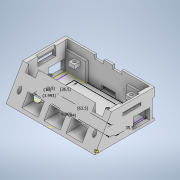
# Autodesk Inventor part: Base Onixium
Saved by Autodesk Inventor 2021 (Build 250183000, 183)
## iProperties
Created: 2021-10-26
Part Number: Base Onixium
Material: Genérico
Document SubType Name: Chapa
Designer: Juan Camilo
Density: 1 g/cm^3
Sheet Metal Rule: Por defecto_mm
Appearance: Valor por defecto
Author: Juan Camilo
Autodesk Inventor part; units mm, degrees
ref_plane "YZ Plane" through (0, 0, 0) normal (1, 0, 0) x (0, 1, 0)
ref_plane "XZ Plane" through (0, 0, 0) normal (0, 1, 0) x (-1, 0, 0)
ref_plane "XY Plane" through (0, 0, 0) normal (0, 0, 1) x (1, 0, 0)
sketch "Boceto2" plane through (0, 0, 0) normal (0, 1, 0) x (-1, 0, 0)
  line L0 (-49, 0) -> (49, 0)
  line L1 (49, 0) -> (49, -87)
  line L2 (49, -87) -> (-49, -87)
  line L3 (-49, -87) -> (-49, 0)
  line L4 (0, -87) -> (0, 0) construction
  circle A0 centre (-41.5, -7.5) radius 1.75
  circle A1 centre (41.5, -7.5) radius 1.75
  line L5 (-26, -87) -> (-26, -66)
  line L6 (-26, -66) -> (-49, -66)
  line L7 (26, -87) -> (26, -66)
  line L8 (26, -66) -> (49, -66)
  line L9 (49, -12) -> (-49, -12) construction
  line L10 (44.5, -24.05) -> (28.5, -24.05)
  line L11 (28.5, -24.05) -> (28.5, -13.05)
  line L12 (28.5, -13.05) -> (44.5, -13.05)
  line L13 (44.5, -13.05) -> (44.5, -24.05)
  line L14 (42.5, -23.55) -> (31.5, -23.55)
  line L15 (31.5, -14.85) -> (42.5, -14.85)
  line L16 (42.5, -14.85) -> (42.5, -23.55)
  circle A2 centre (30.2, -19.25) radius 1.05
  line L17 (31.5, -14.85) -> (31.5, -23.55)
  line L18 (-42.5, -23.55) -> (-31.5, -23.55)
  line L19 (-31.5, -14.85) -> (-42.5, -14.85)
  line L20 (-42.5, -14.85) -> (-42.5, -23.55)
  circle A3 centre (-30.2, -19.25) radius 1.05
  line L21 (-31.5, -14.85) -> (-31.5, -23.55)
  circle A4 centre (13, -21.5) radius 2.5
  circle A5 centre (-13, -21.5) radius 2.5
  circle A6 centre (16, -70) radius 2.5
  circle A7 centre (-16, -70) radius 2.5
  point P0 (26, -87)
  dimension "d6" = 3.5
  dimension "d210" = 0
  dimension "d219" = 87
  dimension "d220" = 21
  dimension "d221" = 12
  dimension "d222" = 23
  dimension "d223" = 98
  dimension "d224" = 7.5
  dimension "d225" = 7.5
  dimension "d226" = 79.5
  dimension "d229" = 2.1
  dimension "d230" = 9
  dimension "d231" = 11
  dimension "d232" = 16
  dimension "d235" = 1
  dimension "d236" = 3.6
  dimension "d239" = 2.1
  dimension "d241" = 1.3
  dimension "d242" = 5
  dimension "d243" = 36
  dimension "d244" = 9.5
  dimension "d245" = 5
  dimension "d246" = 17
  dimension "d247" = 10
  dimension "d252" = 8.7
  dimension "d254" = 4.3
  dimension "d255" = 4
  dimension "d256" = 11
  dimension "d257" = 54
  dimension "d258" = 2.85
  constraints: 44 end point, 10 symmetric about line, 8 centre point, 5 parallel, 5 point on line, 4 horizontal, 4 perpendicular, 3 midpoint, 1 equal radius, 1 vertical, 3 other
  measures "d6" diameter of A0
  measures "d210" distance of point (0, 0) L4.end
  measures "d219" distance of L1.start L1.end
  measures "d220" distance of L7.start L8.start
  measures "d221" distance between parallel lines of L0 L9
  measures "d222" distance of L8.start L8.end
  measures "d223" distance of L0.start L1.start
  measures "d224" distance from line of L1 A1.centre
  measures "d225" distance from line of L0 A1.centre
  measures "d229" diameter of L9 L12
  measures "d230" diameter of L1 L13
  measures "d231" distance of L10.end L11.end
  measures "d232" distance of L10.start L10.end
  measures "d235" diameter of L14 L10
  measures "d236" diameter of L15 L12
  measures "d239" diameter of A2
  measures "d241" distance from line of L17 A2.centre
  measures "d242" diameter of A4
  measures "d243" distance from line of L1 A4.centre
  measures "d244" distance from line of L9 A4.centre
  measures "d245" diameter of A6
  measures "d246" distance from line of L2 A6.centre
  measures "d247" distance from line of L7 A6.centre
  measures "d252" distance of L15.start L14.end
  measures "d254" distance from line of L14 A2.centre
  measures "d255" diameter of L16 L13
  measures "d256" distance of L15.start L15.end
  measures "d257" distance between parallel lines of L9 L8
  measures "d258" distance between parallel lines of L9 L15
extrude "Extrusion Base" add sketch "Boceto2" along normal blind 2 contours L0 L1 L8 L7 L2 L5 L6 L3 | L10 L11 L12 L13
sketch "Boceto4" plane through (-49, 0, -66) normal (-1, 0, 0) x (0, 0, 1)
  line L0 (66, 0) -> (0, 0) projected
  line L1 (66, 0) -> (64.8476, 2)
  line L2 (66, 0) -> (68.3082, 0) construction
  line L3 (64.8476, 2) -> (66, 2)
  line L4 (66, 0) -> (66, 2) projected
  line L5 (66, 2) -> (66, 0)
  dimension "d24" = 119.95
  constraints: 8 end point, 2 horizontal, 1 equal length, 1 perpendicular
  measures "d24" angle of L2 L1
extrude "Extrusión Angulo parte de adelante" cut sketch "Boceto4" against normal blind 100
sketch "Boceto5" plane through (0, 2, 0) normal (0, 1, 0) x (1, 0, 0)
  line L0 (49, 66) -> (26, 66) projected
  line L1 (-49, 66) -> (-49, 1.1524) projected
  line L2 (49, 66) -> (-49, 66)
  line L3 (-49, 66) -> (-49, 61.5)
  line L4 (-49, 61.5) -> (49, 61.5)
  line L5 (49, 61.5) -> (49, 66)
  point P0 (0, 0)
  dimension "d27" = 4.5
  constraints: 8 end point, 2 parallel, 1 horizontal, 1 perpendicular, 1 point on line
  measures "d27" distance of L3.end L2.end
extrude "parte trasera diseño" add sketch "Boceto5" along normal blind 30
sketch "Boceto6" plane through (-26, 0, -66) normal (0, 0, -1) x (-1, 0, 0)
  line L0 (23, 0) -> (23, 32) projected
  line L1 (23, 0) -> (23, 3.33)
  line L2 (23, 3.33) -> (0, 3.33)
  line L3 (0, 3.33) -> (0, 22.33)
  line L4 (0, 22.33) -> (23, 22.33)
  line L5 (23, 22.33) -> (23, 3.33)
  line L6 (-26, 0) -> (-26, 32)
  line L7 (-75, 32) -> (23, 32) projected
  line L8 (-52, 3.33) -> (-52, 22.33)
  line L9 (-52, 22.33) -> (-75, 22.33)
  line L10 (-75, 3.33) -> (-52, 3.33)
  line L11 (-75, 0) -> (-75, 32)
  line L12 (-75, 22.33) -> (-75, 3.33)
  dimension "d30" = 3.33
  dimension "d31" = 23
  dimension "d32" = 19
  constraints: 22 end point, 5 symmetric about line, 2 parallel, 2 point on line, 1 horizontal, 1 midpoint, 1 perpendicular
  measures "d30" distance of L0.start L1.end
  measures "d31" distance of L3.end L4.end
  measures "d32" distance of L2.end L3.end
extrude "Extrusión parte trasera diseño con empalmes" cut sketch "Boceto6" against normal blind 2.5
fillet "Empalme parte trasera diseño" radius 2 4 edges at (-37.5, 22.33, -66) (-37.5, 3.33, -66) (37.5, 3.33, -66) (37.5, 22.33, -66)
sketch "Boceto7" plane through (0, 32, 0) normal (0, 1, 0) x (1, 0, 0)
  line L0 (49, 61.5) -> (49, 66) projected
  line L1 (49, 61.5) -> (22.385, 61.5)
  line L2 (22.385, 61.5) -> (22.385, 64)
  line L3 (22.385, 64) -> (49, 64)
  line L4 (49, 64) -> (49, 61.5)
  line L5 (49, 61.5) -> (-49, 61.5) projected
  line L6 (0, 61.5) -> (0, 0)
  line L7 (-49, 61.5) -> (-49, 66)
  line L8 (-49, 61.5) -> (-22.385, 61.5)
  line L9 (-22.385, 61.5) -> (-22.385, 64)
  line L10 (-22.385, 64) -> (-49, 64)
  line L11 (-22.385, 61.5) -> (22.385, 61.5)
  line L12 (22.385, 61.5) -> (22.385, 64)
  line L13 (22.385, 64) -> (-22.385, 64)
  line L14 (-22.385, 64) -> (-22.385, 61.5)
  dimension "d36" = 26.615
  dimension "d37" = 2.5
  constraints: 26 end point, 4 parallel, 4 symmetric about line, 2 horizontal, 2 perpendicular, 1 midpoint, 1 vertical
  measures "d36" distance of L2.end L3.end
  measures "d37" distance of L1.end L2.end
extrude "Parte delantera de la parte trasera diseño" cut sketch "Boceto7" against normal blind 30 contours L5 L9 L13 L2
sketch "Boceto8" plane through (22.385, 32, -64) normal (-1, 0, 0) x (0, 0, 1)
  line L0 (2.5, 0) -> (2.5, -30) projected
  line L1 (2.5, -30) -> (0, -30)
  line L2 (0, -30) -> (0, -9)
  line L3 (0, -9) -> (2.5, -9)
  line L4 (2.5, -9) -> (2.5, -30)
  line L5 (0, 0) -> (2.5, 0) projected
  line L6 (2.5, -9) -> (0, -9)
  line L7 (0, -9) -> (0, 0)
  line L8 (0, 0) -> (2.5, 0)
  line L9 (2.5, 0) -> (2.5, -9)
  point P0 (64, -32)
  point P1 (0, -9)
  point P2 (2.5, -9)
  dimension "d40" = 2.5
  dimension "d41" = 21
  constraints: 16 end point, 4 parallel, 2 horizontal, 2 perpendicular
  measures "d40" distance of L2.end L3.end
  measures "d41" distance of L1.end L2.end
extrude "Extrusión Parte delantera de la parte trasera del diseño" cut sketch "Boceto8" along normal blind 67.77 and the other way blind 23.15 contours L0 L3 L7 L5
sketch "Boceto9" plane through (0, 32, 0) normal (0, 1, 0) x (1, 0, 0)
  line L0 (49, 0) -> (49, 66) projected
  line L1 (49, 66) -> (15, 66)
  line L2 (49, 66) -> (-49, 66) projected
  line L3 (15, 66) -> (5, 66)
  line L4 (5, 66) -> (5, 64)
  line L5 (5, 64) -> (15, 64)
  line L6 (15, 64) -> (15, 66)
  line L7 (0, 66) -> (0, 64)
  line L8 (-45.385, 64) -> (45.535, 64) projected
  line L9 (-49, 66) -> (49, 66)
  line L10 (-15, 66) -> (-5, 66)
  line L11 (-5, 66) -> (-5, 64)
  line L12 (-5, 64) -> (-15, 64)
  line L13 (-15, 64) -> (-15, 66)
  point P0 (0, 0)
  point P1 (-15, 64)
  point P2 (-5, 64)
  dimension "d46" = 34
  dimension "d47" = 10
  dimension "d48" = 2
  dimension "d49" = 2
  constraints: 22 end point, 6 symmetric about line, 3 point on line, 2 parallel, 1 horizontal, 1 midpoint, 1 perpendicular
  measures "d46" distance of L0.end L1.end
  measures "d47" distance of L5.end L4.end
  measures "d48" distance of L4.end L3.end
  measures "d49" distance of L7.start L7.end
extrude "Extrusión Parte Trasera De la Parte trasera diseño" cut sketch "Boceto9" against normal blind 4 contours L6 L5 L4 L2 | L11 L8 L13 L2
sketch "Boceto10" plane through (49, 0, 0) normal (1, 0, 0) x (0, 0, -1)
  line L0 (0, 0) -> (1.1524, 2) projected
  line L1 (1.1524, 2) -> (0, 2)
  line L2 (61.5, 32) -> (66, 32) projected
  line L3 (0, 2) -> (61.5, 2)
  line L4 (61.5, 2) -> (61.5, 32)
  line L5 (61.5, 32) -> (0, 32)
  line L6 (0, 32) -> (0, 2)
  point P0 (1.1524, 2)
  constraints: 10 end point, 2 horizontal, 2 parallel, 1 perpendicular
extrude "Grado de inclinacion de 60.5 de parte delantera" add sketch "Boceto10" against normal blind 4
sketch "Boceto11" plane through (-49, 0, -66) normal (-1, 0, 0) x (0, 0, 1)
  line L0 (64.8476, 2) -> (4.5, 2) projected
  line L1 (64.8476, 2) -> (66, 2) projected
  line L2 (66, 2) -> (66, 32) projected
  line L3 (66, 32) -> (4.5, 32) projected
  line L4 (4.5, 32) -> (4.5, 23) projected
  line L5 (4.5, 2) -> (4.5, 23) projected
  line L6 (4.5, 2) -> (4.5, 32) projected
  line L7 (66, 2) -> (4.5, 2)
  line L8 (4.5, 2) -> (4.5, 32)
  line L9 (4.5, 32) -> (66, 32)
  line L10 (66, 32) -> (66, 2)
  point P0 (66, 0)
  point P1 (4.5, 2)
  constraints: 8 end point, 2 parallel, 1 horizontal, 1 perpendicular
extrude "Lateral derecha de diseño" add sketch "Boceto11" against normal blind 4
sketch "Boceto12" plane through (0, 32, 0) normal (0, 1, 0) x (1, 0, 0)
  line L0 (45, 0) -> (-45, 0)
  line L1 (-45, 0) -> (-45, 4)
  line L2 (-45, 4) -> (45, 4)
  line L3 (45, 4) -> (45, 0)
  line L4 (0, 4) -> (0, 64)
  line L5 (-5, 64) -> (5, 64) projected
  point P0 (0, 0)
  point P1 (-45, 0)
  point P2 (-49, 0)
  dimension "d56" = 4
  constraints: 10 end point, 2 midpoint, 2 parallel, 1 horizontal, 1 perpendicular
  measures "d56" distance of L0.end L1.end
extrude "Parte delantera diseño" add sketch "Boceto12" against normal blind 30
sketch "Boceto13" plane through (49, 0, 0) normal (1, 0, 0) x (0, 0, -1)
  line L0 (1.1524, 2) -> (0, 0) projected
  line L1 (0, 0) -> (18.438, 32)
  line L2 (0, 32) -> (61.5, 32) projected
  line L3 (0, 0) -> (36.9318, 0) construction
  line L4 (18.438, 32) -> (0, 32)
  line L5 (0, 32) -> (0, 0)
  point P0 (4, 32)
  point P1 (1.1524, 2)
  point P2 (4, 32)
  dimension "d59" = 60.05
  constraints: 8 end point, 1 collinear, 1 equal length, 1 horizontal, 1 perpendicular, 1 point on line
  measures "d59" angle of L3 L1
extrude "Lateral izquierda diseño" cut sketch "Boceto13" against normal blind 103.25
sketch "Boceto14" plane through (26, 0, -66) normal (1, 0, 0) x (0, 0, -1)
  line L0 (21, 2) -> (0, 2) projected
  line L1 (21, 2) -> (19.5, 0)
  line L2 (21, 2) -> (23.5, 2) construction
  line L3 (21, 0) -> (0, 0) projected
  line L4 (19.5, 0) -> (21, 0)
  line L5 (21, 0) -> (21, 2) projected
  line L6 (21, 0) -> (21, 2)
  point P0 (-66, 0)
  point P1 (19.5, 0)
  dimension "d62" = 126.87
  constraints: 8 end point, 1 collinear, 1 equal length, 1 horizontal, 1 perpendicular
  measures "d62" angle of L1 L2
extrude "Extrusion para placa trasera" cut sketch "Boceto14" against normal blind 57.5
sketch "Boceto15" plane through (-45, 0, -66) normal (1, 0, 0) x (0, 0, -1)
  line L0 (-47.562, 32) -> (-66, 0) projected
  line L1 (-66, 0) -> (0, 0) projected
  line L2 (0, 0) -> (0, 1.33) projected
  arc A0 (0, 1.33) -> (-2, 3.33) centre (-2, 1.33) ccw projected
  line L3 (-2, 3.33) -> (-2.5, 3.33) projected
  line L4 (-2.5, 3.33) -> (-2.5, 22.33) projected
  line L5 (-2.5, 22.33) -> (-2, 22.33) projected
  arc A1 (-2, 22.33) -> (0, 24.33) centre (-2, 24.33) ccw projected
  line L6 (0, 24.33) -> (0, 32) projected
  line L7 (0, 32) -> (-47.562, 32) projected
  line L8 (-4.5, 32) -> (-47.562, 32) projected
  line L9 (-47.562, 32) -> (-47.562, 0)
  line L10 (0, 0) -> (-66, 0) projected
  line L11 (-66, 0) -> (-47.562, 32) projected
  line L12 (-66, 0) -> (-47.562, 0)
  line L13 (-66, 0) -> (-47.562, 32)
  constraints: 6 end point, 1 collinear, 1 point on line, 1 vertical
extrude "Extrusion capa parte delantera" add sketch "Boceto15" along normal blind 93 contours L9 L1 L0
sketch "Boceto17" plane through (0, 0, 0) normal (0, -1, 0) x (1, 0, 0)
  line L0 (-49, 0) -> (49, 0) projected
  line L1 (49, 0) -> (41.5, 0)
  line L2 (41.5, 0) -> (41.5, -7.5)
  line L3 (41.5, -7.5) -> (49, -7.5)
  line L4 (49, -7.5) -> (49, 0)
  circle A0 centre (41.5, -7.5) radius 1.75
  line L5 (0, 0) -> (0, -85.5)
  line L6 (-26, -85.5) -> (26, -85.5) projected
  circle A1 centre (-41.5, -7.5) radius 1.75
  dimension "d67" = 7.5
  dimension "d68" = 7.5
  dimension "d69" = 3.5
  constraints: 10 end point, 2 centre point, 2 parallel, 1 coincident, 1 horizontal, 1 midpoint, 1 perpendicular, 1 symmetric about line, 1 other
  measures "d67" distance of L3.end L2.end
  measures "d68" distance of L2.end L1.end
  measures "d69" diameter of A0
extrude "Extrusión huecos tornillos parte delantera" cut sketch "Boceto17" against normal blind 90.25 contours A0 L3 L2 | L2 L3 A0 | A1
sketch "Boceto24" plane through (0, 2, 0) normal (0, 1, 0) x (1, 0, 0)
  line L0 (45.535, 61.5) -> (45, 61.5) projected
  line L1 (45, 61.5) -> (32, 61.5)
  line L2 (32, 61.5) -> (32, 31.5)
  line L3 (32, 31.5) -> (45, 31.5)
  line L4 (45, 31.5) -> (45, 61.5)
  circle A0 centre (32, 31.5) radius 1.75
  circle A1 centre (32, 31.5) radius 2.25
  line L5 (-5, 64) -> (5, 64) projected
  line L6 (0, 64) -> (0, 39.9317)
  circle A2 centre (-32, 31.5) radius 1.75
  circle A3 centre (-32, 31.5) radius 2.25
  point P0 (0, 0)
  dimension "d120" = 13
  dimension "d121" = 30
  dimension "d122" = 3.5
  dimension "d123" = 4.5
  dimension "d143" = 59.5
  constraints: 10 end point, 4 centre point, 3 coincident, 2 parallel, 2 symmetric about line, 1 horizontal, 1 midpoint, 1 perpendicular, 1 vertical, 2 other
  measures "d120" distance of L3.end L2.end
  measures "d121" distance of L2.end L1.end
  measures "d122" diameter of A0
  measures "d123" diameter of A1
extrude "Tornillos Placa" add sketch "Boceto24" along normal blind 18 contours A1 L3 A0 L2 | L2 A0 L3 A1 | A3
thread "Rosca1" size "M3.5x0.6" class "6H" standard "ANSI Metric M Profile" full length
thread "Rosca2" size "M3.5x0.6" class "6H" standard "ANSI Metric M Profile" full length
sketch "Boceto25" plane through (-49, 0, -66) normal (-1, 0, 0) x (0, 0, 1)
  line L0 (5.5, 15) -> (23.5, 15)
  line L1 (23.5, 15) -> (23.5, 3)
  line L2 (23.5, 3) -> (5.5, 3)
  line L3 (5.5, 3) -> (5.5, 15)
  line L4 (2.5, 22.33) -> (2.5, 3.33) projected
  line L5 (0, 0) -> (66, 0) projected
  dimension "d130" = 3
  dimension "d131" = 3
  dimension "d132" = 18
  dimension "d133" = 12
  constraints: 8 end point, 2 parallel, 1 horizontal, 1 perpendicular
  measures "d130" distance between parallel lines of L4 L3
  measures "d131" distance between parallel lines of L5 L2
  measures "d132" distance of L0.start L0.end
  measures "d133" distance of L0.end L1.end
extrude "Extrusión sensores laterales" cut sketch "Boceto25" against normal blind 98.25
sketch "Boceto26" plane through (26, 2, -66) normal (0, 0, -1) x (-1, 0, 0)
  line L0 (18.5, 5) -> (33.5, 5)
  line L1 (33.5, 5) -> (33.5, 0)
  line L2 (33.5, 0) -> (18.5, 0)
  line L3 (18.5, 0) -> (18.5, 5)
  line L4 (52, 0) -> (0, 0) projected
  line L5 (52, 0) -> (52, 22.33) projected
  line L6 (0, 0) -> (0, 22.33) projected
  point P0 (26, -2)
  dimension "d136" = 15
  dimension "d137" = 5
  dimension "d138" = 0
  dimension "d139" = 18.5
  dimension "d140" = 18.5
  constraints: 8 end point, 2 parallel, 1 horizontal, 1 perpendicular
  measures "d136" distance of L0.start L0.end
  measures "d137" distance of L2.end L0.start
  measures "d138" distance between parallel lines of L4 L2
  measures "d139" distance between parallel lines of L5 L1
  measures "d140" distance between parallel lines of L6 L3
extrude "Extrusión agujero cables inferiores" cut sketch "Boceto26" against normal blind 3
sketch "Boceto27" plane through (-45, 2, -18.438) normal (0, 0, -1) x (-1, 0, 0)
  line L0 (-78.5, 13) -> (-60.5, 13)
  line L1 (-60.5, 13) -> (-60.5, 1)
  line L2 (-60.5, 1) -> (-78.5, 1)
  line L3 (-78.5, 1) -> (-78.5, 13)
  line L4 (0, 0) -> (-90, 0) projected
  line L5 (-90, 0) -> (-90, 30) projected
  line L6 (-54.1, 13) -> (-36.1, 13)
  line L7 (-36.1, 13) -> (-36.1, 1)
  line L8 (-36.1, 1) -> (-54.1, 1)
  line L9 (-54.1, 1) -> (-54.1, 13)
  line L10 (-29.7, 13) -> (-11.7, 13)
  line L11 (-11.7, 13) -> (-11.7, 1)
  line L12 (-11.7, 1) -> (-29.7, 1)
  line L13 (-29.7, 1) -> (-29.7, 13)
  point P0 (-45, -2)
  point P1 (-13.5, 0)
  point P2 (-76.5, 0)
  dimension "d144" = 18
  dimension "d145" = 12
  dimension "d146" = 1
  dimension "d147" = 11.5
  dimension "d148" = 1
  dimension "d149" = 12
  dimension "d150" = 18
  dimension "d151" = 6.4
  dimension "d152" = 6.4
  dimension "d153" = 1
  dimension "d154" = 18
  dimension "d155" = 12
  constraints: 24 end point, 6 parallel, 3 horizontal, 3 perpendicular
  measures "d144" distance of L0.start L0.end
  measures "d145" distance of L0.end L1.end
  measures "d146" distance between parallel lines of L4 L2
  measures "d147" distance between parallel lines of L5 L3
  measures "d148" distance between parallel lines of L4 L8
  measures "d149" distance of L8.end L6.start
  measures "d150" distance of L6.start L6.end
  measures "d151" distance between parallel lines of L9 L1
  measures "d152" distance between parallel lines of L7 L13
  measures "d153" distance between parallel lines of L4 L12
  measures "d154" distance of L10.start L10.end
  measures "d155" distance of L10.end L11.end
extrude "Extrusión sensores delanteros" cut sketch "Boceto27" against normal blind 19.25
sketch "Boceto28" plane through (-22.385, 2, -61.5) normal (0, 0, 1) x (1, 0, 0)
  line L0 (-12.615, 14) -> (-5.615, 14)
  line L1 (-5.615, 14) -> (-5.615, 18)
  line L2 (-5.615, 18) -> (-12.615, 18)
  line L3 (-12.615, 18) -> (-12.615, 14)
  line L4 (0, 0) -> (-22.615, 0) projected
  line L5 (-22.615, 21) -> (-22.615, 0) projected
  line L6 (22.385, -2) -> (22.385, 31.9246)
  line L7 (57.385, 14) -> (50.385, 14)
  line L8 (50.385, 14) -> (50.385, 18)
  line L9 (50.385, 18) -> (57.385, 18)
  line L10 (57.385, 18) -> (57.385, 14)
  dimension "d158" = 18
  dimension "d159" = 4
  dimension "d160" = 7
  dimension "d161" = 10
  constraints: 18 end point, 4 symmetric about line, 2 parallel, 1 horizontal, 1 perpendicular, 1 vertical
  measures "d158" distance between parallel lines of L4 L2
  measures "d159" distance between parallel lines of L0 L2
  measures "d160" distance of L1.end L2.end
  measures "d161" distance between parallel lines of L5 L3
extrude "Extrusión pads tornillos traseros placa" add sketch "Boceto28" along normal blind 7
sketch "Boceto29" plane through (-35, 20, -61.5) normal (0, 1, 0) x (1, 0, 0)
  line L0 (7, -7) -> (0, -7) projected
  line L1 (3.5, -7) -> (3.5, 1.276)
  line L2 (0, 0) -> (0, -7) projected
  line L3 (0, -3.5) -> (7, -3.5)
  line L4 (7, 0) -> (7, -7) projected
  circle A0 centre (3.5, -3.5) radius 1.75
  line L5 (35, 2.507) -> (35, -61.5)
  circle A1 centre (66.5, -3.5) radius 1.75
  dimension "d164" = 3.5
  constraints: 6 end point, 4 midpoint, 2 centre point, 2 vertical, 1 symmetric about line, 1 other
  measures "d164" diameter of A0
extrude "Extrusión tornillos" cut sketch "Boceto29" against normal blind 4.75 contours A0 L3 L1 | L1 L3 A0 | L3 L1 A0 | L3 A0 L1 | A1
sketch "Boceto placa" plane through (0, 2, 0) normal (0, 1, 0) x (1, 0, 0)
  circle A0 centre (-32, 31.5) radius 1.75 projected
  circle A1 centre (31.5, 58) radius 1.75 projected
  line L0 (-32, 31.5) -> (31.5, 31.5)
  line L1 (31.5, 31.5) -> (31.5, 58)
  line L2 (31.5, 58) -> (-32, 58)
  line L3 (-32, 58) -> (-32, 31.5)
  line L4 (-42, 27.507) -> (42, 27.507)
  line L5 (42, 27.507) -> (42, 63.007)
  line L6 (42, 63.007) -> (-42, 63.007)
  line L7 (-42, 63.007) -> (-42, 27.507)
  line L8 (-45, 61.5) -> (-45, 18.438) projected
  line L9 (45, 18.438) -> (45, 61.5) projected
  line L10 (-22.385, 61.5) -> (-45, 61.5) projected
  line L11 (-44, 25.3) -> (-33.55, 25.3) projected
  line L12 (-45, 18.438) -> (45, 18.438) projected
  point P0 (0, 0)
  dimension "d167" = 63.5
  dimension "d168" = 26.5
  dimension "d172" = 84
  dimension "d176" = 10
  dimension "d177" = 3.993
  dimension "d178" = 3.5
  dimension "d179" = 35.5
  dimension "d180" = 9.069
  constraints: 16 end point, 4 parallel, 2 horizontal, 2 perpendicular
  measures "d167" distance of L0.start L0.end
  measures "d168" distance of L2.end L0.start
  measures "d172" distance of L4.start L4.end
  measures "d176" distance from line of L7 L0.start
  measures "d177" distance from line of L4 L0.start
  measures "d178" diameter of A0
  measures "d179" distance between parallel lines of L6 L4
  measures "d180" distance between parallel lines of L12 L4
sketch "Boceto32" plane through (0, 32, 0) normal (0, 1, 0) x (1, 0, 0)
  line L0 (45, 31) -> (47, 31)
  line L1 (47, 31) -> (47, 51)
  line L2 (47, 51) -> (45, 51)
  line L3 (45, 51) -> (45, 31)
  line L4 (49, 66) -> (15, 66) projected
  line L5 (45, 18.438) -> (49, 18.438) projected
  line L6 (49, 66) -> (49, 18.438) projected
  line L7 (0, 0) -> (0, 66)
  line L8 (5, 66) -> (-5, 66) projected
  line L9 (-45, 31) -> (-47, 31)
  line L10 (-47, 31) -> (-47, 51)
  line L11 (-47, 51) -> (-45, 51)
  line L12 (-45, 51) -> (-45, 31)
  dimension "d181" = 15
  dimension "d182" = 20
  dimension "d183" = 12.562
  dimension "d184" = 2
  dimension "d185" = 2
  constraints: 18 end point, 4 symmetric about line, 2 parallel, 1 horizontal, 1 midpoint, 1 perpendicular
  measures "d181" distance between parallel lines of L4 L2
  measures "d182" distance of L2.end L0.start
  measures "d183" distance between parallel lines of L5 L0
  measures "d184" distance of L1.end L2.end
  measures "d185" distance between parallel lines of L6 L1
extrude "Extrusión24" cut sketch "Boceto32" against normal blind 10
sketch "Boceto33" plane through (49, 0, 0) normal (1, 0, 0) x (0, 0, -1)
  line L0 (51, 25) -> (31, 25)
  line L1 (31, 25) -> (31, 22)
  line L2 (31, 22) -> (51, 22)
  line L3 (51, 22) -> (51, 25)
  line L4 (51, 22) -> (31, 22) projected
  line L5 (31, 32) -> (31, 22) projected
  line L6 (51, 32) -> (51, 22) projected
  point P0 (0, 0)
  dimension "d188" = 0
  dimension "d189" = 0
  dimension "d190" = 3
  dimension "d191" = 0
  constraints: 8 end point, 2 parallel, 1 horizontal, 1 perpendicular
  measures "d188" distance between parallel lines of L4 L2
  measures "d189" distance between parallel lines of L5 L1
  measures "d190" distance between parallel lines of L2 L0
  measures "d191" distance between parallel lines of L6 L3
extrude "Extrusión25" cut sketch "Boceto33" against normal blind 123.5
sketch "Boceto34" plane through (49, 22, -31) normal (0, 0, -1) x (-1, 0, 0)
  line L0 (0, 0) -> (4, 0)
  line L1 (4, 0) -> (4, 10)
  line L2 (4, 10) -> (-1.4435, 0)
  line L3 (-1.4435, 0) -> (4, 0)
  line L4 (0, 10) -> (0, -22) projected
  line L5 (49, -22) -> (49, 0)
  line L6 (98, 0) -> (94, 0)
  line L7 (94, 0) -> (94, 10)
  line L8 (94, 10) -> (99.4435, 0)
  line L9 (99.4435, 0) -> (98, 0)
  constraints: 18 end point, 4 symmetric about line, 2 vertical, 1 perpendicular
extrude "Extrusión26" cut sketch "Boceto34" along normal blind 20
sketch "Boceto36" plane through (0, 2, 0) normal (0, 1, 0) x (1, 0, 0)
  line L0 (-32, 28.938) -> (32, 28.938)
  line L1 (32, 28.938) -> (32, 27.938)
  line L2 (32, 27.938) -> (-32, 27.938)
  line L3 (-32, 27.938) -> (-32, 28.938)
  line L4 (-45, 31) -> (-45, 51) projected
  line L5 (45, 51) -> (45, 31) projected
  line L6 (-45, 18.438) -> (45, 18.438) projected
  point P0 (0, 0)
  dimension "d198" = 13
  dimension "d199" = 64
  dimension "d200" = 13
  dimension "d201" = 1
  dimension "d202" = 9.5
  constraints: 8 end point, 2 parallel, 1 horizontal, 1 perpendicular
  measures "d198" distance between parallel lines of L4 L3
  measures "d199" distance of L1.end L2.end
  measures "d200" distance between parallel lines of L5 L1
  measures "d201" distance between parallel lines of L2 L0
  measures "d202" distance between parallel lines of L6 L2
extrude "Extrusión pared bateria" add sketch "Boceto36" along normal blind 7
sketch "Boceto39" plane through (0, 2, 0) normal (0, 1, 0) x (1, 0, 0)
  line L0 (-42.5, 23.55) -> (-31.5, 23.55)
  line L1 (-31.5, 23.55) -> (-31.5, 14.8119)
  line L2 (-31.5, 14.8119) -> (-42.5, 14.8119)
  line L3 (-42.5, 14.8119) -> (-42.5, 23.55)
  circle A0 centre (-30.2, 19.25) radius 1.1
  line L4 (-7.5, 64) -> (7.5, 64) projected
  line L5 (0, 64) -> (0, 18.438)
  line L6 (-29.5343, 18.438) -> (29.5343, 18.438) projected
  line L7 (42.5, 23.55) -> (31.5, 23.55)
  line L8 (31.5, 23.55) -> (31.5, 14.8119)
  line L9 (31.5, 14.8119) -> (42.5, 14.8119)
  line L10 (42.5, 14.8119) -> (42.5, 23.55)
  circle A1 centre (30.2, 19.25) radius 1.1
  arc A2 (-29.5343, 18.438) -> (-30.8657, 18.438) centre (-30.2, 19.25) ccw projected
  point P0 (0, 0)
  dimension "d259" = 11
  dimension "d262" = 2.2
  dimension "d263" = 1.3
  dimension "d264" = 4.3
  dimension "d270" = 2.15
  constraints: 18 end point, 5 symmetric about line, 2 centre point, 2 midpoint, 2 parallel, 1 horizontal, 1 perpendicular, 1 other
  measures "d259" distance of L0.start L0.end
  measures "d262" diameter of A0
  measures "d263" distance from line of L1 A0.centre
  measures "d264" distance from line of L0 A0.centre
extrude "Extrusión arreglo sensores" cut sketch "Boceto39" along normal mid plane 85.25
sketch "Boceto40" plane through (0, 2, 0) normal (0, 1, 0) x (1, 0, 0)
  line L0 (-30.65, 14.8119) -> (-31.5, 14.8119)
  line L1 (-5, 64) -> (5, 64) projected
  line L2 (0, 64) -> (0, 18.438)
  line L3 (-29.5343, 18.438) -> (29.5343, 18.438) projected
  line L4 (31.5, 23.55) -> (31.5, 14.8119)
  line L5 (31.5, 23.55) -> (30.65, 23.55)
  line L6 (30.65, 23.55) -> (30.65, 14.8119)
  line L7 (30.65, 14.8119) -> (31.5, 14.8119)
  line L8 (-31.5, 23.55) -> (-28.1, 23.55)
  line L9 (-28.1, 23.55) -> (-28.1, 14.8119)
  line L10 (-28.1, 14.8119) -> (-31.5, 14.8119)
  line L11 (-31.5, 14.8119) -> (-31.5, 23.55)
  arc A0 (-29.4579, 18.438) -> (-30.9421, 18.438) centre (-30.2, 19.25) ccw projected
  line L12 (31.5, 23.55) -> (28.1, 23.55)
  line L13 (28.1, 23.55) -> (28.1, 14.8119)
  line L14 (28.1, 14.8119) -> (31.5, 14.8119)
  line L15 (31.5, 14.8119) -> (31.5, 23.55)
  point P0 (0, 0)
  point P1 (-31.5, 14.8119)
  point P2 (31.5, 14.8119)
  dimension "d271" = 1
  constraints: 28 end point, 7 symmetric about line, 2 midpoint, 2 parallel, 1 horizontal, 1 perpendicular
  measures "d271" distance edge to line of A0 L9
extrude "Extrusión desnivel sensores" cut sketch "Boceto40" along normal mid plane 2
equation "\"Radio_pliegue\" = Grosor"
equation "\"Anchura_desahogo_plegado\" = Grosor"
equation "\"Profundidad_desahogo_plegado\" = 0.5 * Grosor"
equation "\"Tamaño_destalonado\" = 4 * Grosor"
equation "\"Remanente_mínimo\" = 2 * Grosor"
equation "\"Radiodetransición\" = Radio_pliegue"
equation "\"Tamaño_de_radio_de_Jacobi\" = Radio_pliegue"
equation "\"TamañoSeparación\" = Grosor"
equation "\"Grosor\" = 0.5"
